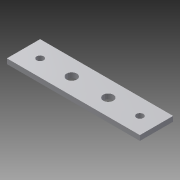
# Autodesk Inventor part: Part1
Saved by Autodesk Inventor 2015 (Build 190159000, 159)
## iProperties
Created: 2015-06-23
Part Number: Part1
Material: アルミニウム 5052 H32
Document SubType Name: Modeling
Designer: kenta
Density: 2.68 g/cm^3
Appearance: サテン
Author: kenta
Autodesk Inventor part; units mm, degrees
ref_plane "YZ Plane" through (0, 0, 0) normal (1, 0, 0) x (0, 1, 0)
ref_plane "XZ Plane" through (0, 0, 0) normal (0, 1, 0) x (-1, 0, 0)
ref_plane "XY Plane" through (0, 0, 0) normal (0, 0, 1) x (1, 0, 0)
sketch "スケッチ1" plane through (0, 0, 0) normal (0, 0, 1) x (1, 0, 0)
  line L0 (-20, 5) -> (20, 5)
  line L1 (20, 5) -> (20, -5)
  line L2 (20, -5) -> (-20, -5)
  line L3 (-20, -5) -> (-20, 5)
  line L4 (-20, 5) -> (20, -5) construction
  line L5 (20, 5) -> (-20, -5) construction
  point P0 (0, 0)
  dimension "d0" = 40
  dimension "d1" = 10
  constraints: 12 end point, 2 midpoint, 2 parallel, 1 horizontal, 1 perpendicular
  measures "d0" distance of L1.end L2.end
  measures "d1" distance of L0.end L1.end
extrude "押し出し1" add sketch "スケッチ1" along normal blind 1.5
sketch "スケッチ2" plane through (0, 0, 1.5) normal (0, 0, 1) x (1, 0, 0)
  point P0 (0, 0)
  point P1 (-5.5, 0)
  point P2 (5.5, 0)
  dimension "d4" = 0
  dimension "d5" = 11
  dimension "d6" = 5.5
  constraints: 1 horizontal alignment
  measures "d4" vertical distance of point (0, 0) point (-5.5, 0)
  measures "d5" distance of point (5.5, 0) point (-5.5, 0)
  measures "d6" distance of point (-5.5, 0) point (0, 0)
hole "穴1" at (-5.5, 0, 1.5) at (5.5, 0, 1.5) direction (0, 0, -1) diameter 3.1 end through all
sketch "スケッチ3" plane through (0, 0, 1.5) normal (0, 0, 1) x (1, 0, 0)
  line L0 (20, -5) -> (20, 5) projected
  line L1 (-20, 5) -> (-20, -5) projected
  point P0 (0, 0)
  point P1 (-15, 0)
  point P2 (15, 0)
  dimension "d14" = 5
  dimension "d15" = 5
  measures "d14" distance from line of point (15, 0) L0
  measures "d15" distance from line of point (-15, 0) L1
hole "穴2" at (-15, 0, 1.5) at (15, 0, 1.5) direction (0, 0, -1) diameter 2.1 end through all
